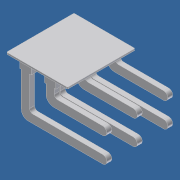
# Autodesk Inventor part: M202830_terminal_angW
Saved by Autodesk Inventor 2014 (Build 180170000, 170)
## iProperties
Category: PARTsolutions
Created: 2013-12-29
Part Number: M202830_terminal_angW
Catalog Web Link: www.cadenas.de
Description: Angle Mount Miniature Toggles-terminals - Series M - Miniature Toggles
Document SubType Name: Modeling
Designer: PARTsolutions
Material: Generic
Density: 1 g/cm^3
Appearance: RGB(192,192,192)
NB: M202830_terminal_angW
NN: Angle Mount Miniature Toggles-terminals
NT: Series M - Miniature Toggles
NBSYN: $PN.$CMR.
LINA: M202830_terminal_angW
PN: M202830_terminal_ang
SRS: M20
PLS: 2
CRCTSALG: '2','2 - ON/NONE/ON','3','3 - ON/OFF/ON','5','5 - ON/NONE/(ON)','8','8 - (ON)/OFF/(ON)','9','9 - ON/OFF/(ON)','4', '4 - ON/ON/ON','6','6 - (ON)/ON/(ON)','7','7 - ON/ON/(ON)'
CRCTS: 8
TRMNLSALG: '01','01 - Solder Lug','02','02 - Quick Connect','03','03 - .250" (6.35mm) Straight PC','05', '05 - .425" (10.8mm) Wirewrap','06', '06 - .750" (19.05mm) Wirewrap','07', '07 - .964" (24.5mm) Wirewrap','08', '08 - 1.062" (27.0mm) Wirewrap'
TRMNLS: 30
WIDTH: 0.512
HEIGHT: 0.370
LENGTH: 0.500
A: 0.000
TRMNLNOH: 2.000
POS: 0.095
TRMNLOV: 3.000
D: 0.040
D2: -0.11000
M: 0.09450
NUM: 1.00000
TYPE: 0.10000
DSA: 1.00000
CMR: W
CLR: 0.753,0.753,0.753,0.00
TD: 0.10000
KT: DUMMY
SUPPLIER: NKKSWITCHES
ARTICLENO: M202830_terminal_angW
BOMINFO: M202830_terminal_angW
CREATOR: CADENAS GmbH
PSOL_IDENT_0: {$CADENAS_DATA\23d-libs\nkkswitches\toggle\m\parts\m_ang_t_terminal.prj},237 {VTYP=3D},{NB=M202830_t
PSOL_IDENT_1: erminal_angW},{LINA=M202830_terminal_angW},{NN=Angle Mount Miniature Toggles-terminals},{DATE=02.06.
PSOL_IDENT_2: 2007 15:25:20},{GEOMDATE=02.06.2007 00:00:00},{VERSION=},{LINEID=10},{LINESUBID=-1},{WBVAR=PLS,CRCTS
PSOL_IDENT_3: ,TRMNLS,CMR}  {NB=M202830_terminal_angW},{LINA=M202830_terminal_angW},{KT=DUMMY},{PN=M202830_termina
PSOL_IDENT_4: l_ang},{SRS=M20},{PLS=2},{CRCTSALG='2','2 - ON/NONE/ON','3','3 - ON/OFF/ON','5','5 - ON/NONE/(ON)','
PSOL_IDENT_5: 8','8 - (ON)/OFF/(ON)','9','9 - ON/OFF/(ON)','4', '4 - ON/ON/ON','6','6 - (ON)/ON/(ON)','7','7 - ON/
PSOL_IDENT_6: ON/(ON)'},{CRCTS=8},{TRMNLSALG='01','01 - Solder Lug','02','02 - Quick Connect','03','03 - .250\" (6
PSOL_IDENT_7: .35mm) Straight PC','05', '05 - .425\" (10.8mm) Wirewrap','06', '06 - .750\" (19.05mm) Wirewrap','07
PSOL_IDENT_8: ', '07 - .964\" (24.5mm) Wirewrap','08', '08 - 1.062\" (27.0mm) Wirewrap'},{TRMNLS=30},{WIDTH=0.512}
PSOL_IDENT_9: ,{HEIGHT=0.37},{LENGTH=0.5},{A=0},{TRMNLNOH=2},{POS=0.0945},{TRMNLOV=3},{D=0.04},{D2=-0.11000},{M=0.
PSOL_IDENT_10: 09450},{NUM=1.00000},{TYPE=0.10000},{DSA=1.00000},{CMR=W},{CLR=0.753,0.753,0.753,0.00},{TD=0.10000}
Title: M202830_terminal_angW
Author: Cadenas PARTsolutions
Comments: Series M - Miniature Toggles
Autodesk Inventor part; units mm, degrees
sketch "Sketch_2" plane through (0, 0, 0) normal (0, 1, 0) x (-1, 0, 0)
  line L0 (4.7037, -5.0719) -> (4.7037, 5.0719)
  arc A0 (4.7037, 5.0719) -> (4.5737, 5.2019) centre (4.5737, 5.0719) ccw
  line L1 (4.5737, 5.2019) -> (-4.5737, 5.2019)
  arc A1 (-4.5737, 5.2019) -> (-4.7037, 5.0719) centre (-4.5737, 5.0719) ccw
  line L2 (-4.7037, 5.0719) -> (-4.7037, -5.0719)
  arc A2 (-4.7037, -5.0719) -> (-4.5737, -5.2019) centre (-4.5737, -5.0719) ccw
  line L3 (-4.5737, -5.2019) -> (4.5737, -5.2019)
  arc A3 (4.5737, -5.2019) -> (4.7037, -5.0719) centre (4.5737, -5.0719) ccw
  constraints: 8 end point, 8 point on circle, 4 centre point
extrude "Extrusion1" add sketch "Sketch_2" along normal blind 0.254
sketch "Sketch_1" plane through (0, 0, -4.699) normal (0, 0, 1) x (1, 0, 0)
  line L0 (1.016, 0) -> (1.016, -1.016)
  line L1 (1.016, -1.016) -> (1.27, -1.016)
  line L2 (1.27, -1.016) -> (1.27, -2.4384)
  arc A0 (1.27, -2.4384) -> (2.413, -3.5814) centre (2.413, -2.4384) ccw
  line L3 (2.413, -3.5814) -> (10.0076, -3.5814)
  arc A1 (10.0076, -3.5814) -> (10.0076, -2.3114) centre (10.0076, -2.9464) ccw
  line L4 (10.0076, -2.3114) -> (3.048, -2.3114)
  arc A2 (2.54, -1.8034) -> (3.048, -2.3114) centre (3.048, -1.8034) ccw
  line L5 (2.54, -1.8034) -> (2.54, -1.016)
  line L6 (2.54, -1.016) -> (2.794, -1.016)
  line L7 (2.794, -1.016) -> (2.794, 0)
  line L8 (2.794, 0) -> (1.016, 0)
  constraints: 18 end point, 6 point on circle, 3 centre point
extrude "Extrusion2" add sketch "Sketch_1" along normal mid plane 0.762
pattern_linear "Rectangular Pattern1" count 3 spacing 4.699 along (0, 0, 1) of "Extrusion2"
sketch "Sketch_18" plane through (0, 0, -4.699) normal (0, 0, 1) x (1, 0, 0)
  line L0 (-2.794, 0) -> (-2.794, -1.016)
  line L1 (-2.794, -1.016) -> (-2.54, -1.016)
  line L2 (-2.54, -1.016) -> (-2.54, -6.3754)
  arc A0 (-2.54, -6.3754) -> (-1.524, -7.3914) centre (-1.524, -6.3754) ccw
  line L3 (-1.524, -7.3914) -> (10.0076, -7.3914)
  arc A1 (10.0076, -7.3914) -> (10.0076, -6.1214) centre (10.0076, -6.7564) ccw
  line L4 (10.0076, -6.1214) -> (-0.762, -6.1214)
  arc A2 (-1.27, -5.6134) -> (-0.762, -6.1214) centre (-0.762, -5.6134) ccw
  line L5 (-1.27, -5.6134) -> (-1.27, -1.016)
  line L6 (-1.27, -1.016) -> (-1.016, -1.016)
  line L7 (-1.016, -1.016) -> (-1.016, 0)
  line L8 (-1.016, 0) -> (-2.794, 0)
  constraints: 18 end point, 6 point on circle, 3 centre point
extrude "Extrusion3" add sketch "Sketch_18" along normal mid plane 0.762
pattern_linear "Rectangular Pattern2" count 3 spacing 4.699 along (0, 0, 1) of "Extrusion3"
ref_plane "to_base_XY" through (0, -0.0254, 0) normal (0, 1, 0) x (1, 0, 0)
ref_plane "to_base_YZ" through (0, -0.0254, 0) normal (1, 0, 0) x (0, 0, -1)
ref_plane "to_base_ZX" through (0, -0.0254, 0) normal (0, 0, -1) x (0, 1, 0)
body "Solid1"
